7dba4f9f-154c-4f98-b316-e180ac600f7a (Autodesk Fusion 360 design; units mm, degrees)
Autodesk Fusion 360 part; units mm, degrees
sketch "Sketch1" plane through (0, 0, 0) normal (0, 0, 1) x (1, 0, 0)
  circle A0 centre (0, 0) radius 12.7
  circle A1 centre (0, 0) radius 15.875
  dimension "d1" = 25.4
  dimension "d2" = 31.75
  measures "d1" diameter of A0
  measures "d2" diameter of A1
extrude "Extrude1" add sketch "Sketch1" along normal blind 38.1
sketch "Sketch2" plane through (0, 0, 0) normal (0, 0, -1) x (-1, 0, 0)
  circle A0 centre (0, 0) radius 15.875
  circle A1 centre (0, 0) radius 19.05
  circle A2 centre (0, 0) radius 12.7
  dimension "d5" = 38.1
  measures "d5" diameter of A1
extrude "Extrude2" add sketch "Sketch2" against normal blind 3.175 contours A1
equation "d1 = Shaft_ID"
equation "d2 = Housing_ID"
equation "d3 = Length"
equation "d5 = Flange_OD"
equation "d6 = FlangeT"
equation "Shaft_ID = 1 in"
equation "Housing_ID = 1 1/4\""
equation "FlangeT = ( -1 / 8 ) * 1 in"
equation "Length = 1 1/2\""
equation "Flange_OD = 1 1/2\""
